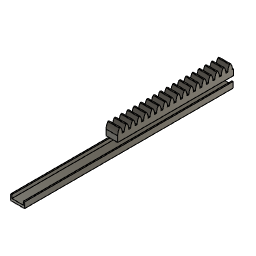
Planar joint (Autodesk Fusion 360 design; units mm, degrees)
Autodesk Fusion 360 part; units mm, degrees
sketch "Sketch1" plane through (0, 0, 0) normal (1, 0, 0) x (0, 1, 0)
  line L0 (0, 0) -> (200, 0)
  line L1 (200, 0) -> (200, 10)
  line L2 (0, 10) -> (0, 0)
  line L3 (0, 15) -> (200, 15.0001) construction
  arc A0 (3.0334, 20) -> (0, 10) centre (18, 10) ccw
  line L4 (3.0334, 20) -> (5.0334, 20)
  line L5 (4.0334, 20) -> (4.0334, 10) construction
  arc A1 (8.0667, 10) -> (5.0334, 20) centre (-9.9333, 10) ccw
  line L6 (14.2098, 20) -> (16.2098, 20)
  line L7 (15.2098, 20) -> (15.2098, 10) construction
  arc A2 (14.2098, 20) -> (11.1765, 10) centre (29.1765, 10) ccw
  arc A3 (19.2432, 10) -> (16.2098, 20) centre (1.2432, 10) ccw
  line L8 (25.3863, 20) -> (27.3863, 20)
  line L9 (26.3863, 20) -> (26.3863, 10) construction
  arc A4 (25.3863, 20) -> (22.3529, 10) centre (40.3529, 10) ccw
  arc A5 (30.4197, 10) -> (27.3863, 20) centre (12.4197, 10) ccw
  line L10 (36.5628, 20) -> (38.5628, 20)
  line L11 (37.5628, 20) -> (37.5628, 10) construction
  arc A6 (36.5628, 20) -> (33.5294, 10) centre (51.5294, 10) ccw
  arc A7 (41.5961, 10) -> (38.5628, 20) centre (23.5961, 10) ccw
  line L12 (47.7392, 20) -> (49.7392, 20)
  line L13 (48.7392, 20) -> (48.7392, 10) construction
  arc A8 (47.7392, 20) -> (44.7059, 10) centre (62.7059, 10) ccw
  arc A9 (52.7726, 10) -> (49.7392, 20) centre (34.7726, 10) ccw
  line L14 (58.9157, 20) -> (60.9157, 20)
  line L15 (59.9157, 20) -> (59.9157, 10) construction
  arc A10 (58.9157, 20) -> (55.8823, 10) centre (73.8823, 10) ccw
  arc A11 (63.9491, 10) -> (60.9157, 20) centre (45.9491, 10) ccw
  line L16 (70.0922, 20) -> (72.0922, 20)
  line L17 (71.0922, 20) -> (71.0922, 10) construction
  arc A12 (70.0922, 20) -> (67.0588, 10) centre (85.0588, 10) ccw
  arc A13 (75.1255, 10) -> (72.0922, 20) centre (57.1255, 10) ccw
  line L18 (81.2687, 20) -> (83.2687, 20)
  line L19 (82.2687, 20) -> (82.2687, 10) construction
  arc A14 (81.2687, 20) -> (78.2353, 10) centre (96.2353, 10) ccw
  arc A15 (86.302, 10) -> (83.2687, 20) centre (68.302, 10) ccw
  line L20 (92.4451, 20) -> (94.4451, 20)
  line L21 (93.4451, 20) -> (93.4451, 10) construction
  arc A16 (92.4451, 20) -> (89.4118, 10) centre (107.4118, 10) ccw
  arc A17 (97.4785, 10) -> (94.4451, 20) centre (79.4785, 10) ccw
  line L22 (103.6216, 20) -> (105.6216, 20)
  line L23 (104.6216, 20) -> (104.6216, 10) construction
  arc A18 (103.6216, 20) -> (100.5882, 10) centre (118.5882, 10) ccw
  arc A19 (108.655, 10) -> (105.6216, 20) centre (90.655, 10) ccw
  line L24 (114.7981, 20) -> (116.7981, 20)
  line L25 (115.7981, 20) -> (115.7981, 10) construction
  arc A20 (114.7981, 20) -> (111.7647, 10) centre (129.7647, 10) ccw
  arc A21 (119.8314, 10) -> (116.7981, 20) centre (101.8314, 10) ccw
  line L26 (125.9745, 20) -> (127.9745, 20)
  line L27 (126.9745, 20) -> (126.9745, 10) construction
  arc A22 (125.9745, 20) -> (122.9412, 10) centre (140.9412, 10) ccw
  arc A23 (131.0079, 10) -> (127.9745, 20) centre (113.0079, 10) ccw
  line L28 (137.151, 20) -> (139.151, 20)
  line L29 (138.151, 20) -> (138.151, 10) construction
  arc A24 (137.151, 20) -> (134.1176, 10) centre (152.1176, 10) ccw
  arc A25 (142.1844, 10) -> (139.151, 20) centre (124.1844, 10) ccw
  line L30 (148.3275, 20) -> (150.3275, 20)
  line L31 (149.3275, 20) -> (149.3275, 10) construction
  arc A26 (148.3275, 20) -> (145.2941, 10) centre (163.2941, 10) ccw
  arc A27 (153.3608, 10) -> (150.3275, 20) centre (135.3608, 10) ccw
  line L32 (159.5039, 20) -> (161.5039, 20)
  line L33 (160.5039, 20) -> (160.5039, 10) construction
  arc A28 (159.5039, 20) -> (156.4706, 10) centre (174.4706, 10) ccw
  arc A29 (164.5373, 10) -> (161.5039, 20) centre (146.5373, 10) ccw
  line L34 (170.6804, 20) -> (172.6804, 20)
  line L35 (171.6804, 20) -> (171.6804, 10) construction
  arc A30 (170.6804, 20) -> (167.6471, 10) centre (185.6471, 10) ccw
  arc A31 (175.7138, 10) -> (172.6804, 20) centre (157.7138, 10) ccw
  line L36 (181.8569, 20) -> (183.8569, 20)
  line L37 (182.8569, 20) -> (182.8569, 10) construction
  arc A32 (181.8569, 20) -> (178.8235, 10) centre (196.8235, 10) ccw
  arc A33 (186.8902, 10) -> (183.8569, 20) centre (168.8902, 10) ccw
  line L38 (193.0334, 20) -> (195.0334, 20)
  line L39 (194.0334, 20) -> (194.0334, 10) construction
  arc A34 (193.0334, 20) -> (190, 10) centre (208, 10) ccw
  arc A35 (198.0667, 10) -> (195.0334, 20) centre (180.0667, 10) ccw
  arc A36 (36.5764, 129.9483) -> (33.491, 119.9458) centre (51.4908, 119.8706) ccw
  arc A37 (41.6234, 119.9458) -> (38.5764, 129.9431) centre (23.4014, 119.855) ccw
  line L40 (37.5764, 129.9457) -> (37.5357, 119.9458) construction
  line L41 (36.5764, 129.9483) -> (38.5764, 129.9431)
  line L42 (182.8569, 170) -> (182.8569, 160) construction
  line L43 (181.8569, 170) -> (183.8569, 170)
  arc A38 (186.8902, 160) -> (183.8569, 170) centre (168.8902, 160) ccw
  arc A39 (181.8569, 170) -> (178.8235, 160) centre (196.8235, 160) ccw
  arc A40 (169.119, 168.7106) -> (167.8682, 158.3358) centre (185.5948, 161.4615) ccw
  line L44 (169.119, 168.7106) -> (171.0886, 169.0579)
  arc A41 (175.8124, 159.7366) -> (171.0886, 169.0579) centre (158.0859, 156.6109) ccw
  line L45 (170.1038, 168.8843) -> (171.8403, 159.0362) construction
  arc A42 (156.7986, 165.2289) -> (157.3684, 154.7945) centre (174.2828, 160.9509) ccw
  line L46 (156.7986, 165.2289) -> (158.678, 165.9129)
  arc A43 (164.9486, 157.5535) -> (158.678, 165.9129) centre (148.0341, 151.3971) ccw
  line L47 (157.7383, 165.5709) -> (161.1585, 156.174) construction
  arc A44 (145.2699, 159.6606) -> (147.6429, 149.4837) centre (163.2314, 158.4837) ccw
  line L48 (145.2699, 159.6606) -> (147.002, 160.6606)
  arc A45 (154.6289, 153.5171) -> (147.002, 160.6606) centre (139.0405, 144.5171) ccw
  line L49 (146.1359, 160.1606) -> (151.1359, 151.5004) construction
  arc A46 (134.8833, 152.1751) -> (138.9875, 142.5648) centre (152.7763, 154.135) ccw
  line L50 (134.8833, 152.1751) -> (136.4154, 153.4606)
  arc A47 (145.1669, 147.75) -> (136.4154, 153.4606) centre (131.3781, 136.1798) ccw
  line L51 (135.6493, 152.8179) -> (142.0772, 145.1574) construction
  arc A48 (125.9543, 142.9996) -> (131.665, 134.248) centre (143.2351, 148.0368) ccw
  line L52 (125.9543, 142.9996) -> (127.2399, 144.5317)
  arc A49 (136.8502, 140.4275) -> (127.2399, 144.5317) centre (125.28, 126.6387) ccw
  line L53 (126.5971, 143.7656) -> (134.2576, 137.3378) construction
  arc A50 (118.7543, 132.413) -> (125.8979, 124.786) centre (134.8979, 140.3745) ccw
  line L54 (118.7543, 132.413) -> (119.7543, 134.1451)
  arc A51 (129.9313, 131.772) -> (119.7543, 134.1451) centre (120.9312, 116.1836) ccw
  line L55 (119.2543, 133.279) -> (127.9146, 128.279) construction
  arc A52 (113.502, 120.737) -> (121.8615, 114.4664) centre (128.0178, 131.3808) ccw
  line L56 (113.502, 120.737) -> (114.1861, 122.6164)
  arc A53 (124.6205, 122.0466) -> (114.1861, 122.6164) centre (118.4641, 105.1322) ccw
  line L57 (113.8441, 121.6767) -> (123.241, 118.2565) construction
  arc A54 (110.3571, 108.3263) -> (119.6784, 103.6026) centre (122.8041, 121.3291) ccw
  line L58 (110.3571, 108.3263) -> (110.7044, 110.2959)
  arc A55 (121.0792, 111.5467) -> (110.7044, 110.2959) centre (117.9535, 93.8202) ccw
  line L59 (110.5307, 109.3111) -> (120.3788, 107.5747) construction
  arc A56 (109.415, 95.5581) -> (119.415, 92.5247) centre (119.415, 110.5247) ccw
  line L60 (109.415, 95.5581) -> (109.415, 97.5581)
  arc A57 (119.415, 100.5914) -> (109.415, 97.5581) centre (119.415, 82.5914) ccw
  line L61 (109.415, 96.5581) -> (119.415, 96.5581) construction
  arc A58 (110.7044, 82.8202) -> (121.0792, 81.5694) centre (117.9535, 99.296) ccw
  line L62 (110.7044, 82.8202) -> (110.3571, 84.7898)
  arc A59 (119.6784, 89.5136) -> (110.3571, 84.7898) centre (122.8041, 71.7871) ccw
  line L63 (110.5307, 83.805) -> (120.3788, 85.5415) construction
  arc A60 (114.1861, 70.4998) -> (124.6205, 71.0695) centre (118.4641, 87.984) ccw
  line L64 (114.1861, 70.4998) -> (113.502, 72.3792)
  arc A61 (121.8615, 78.6498) -> (113.502, 72.3792) centre (128.0178, 61.7353) ccw
  line L65 (113.8441, 71.4395) -> (123.241, 74.8597) construction
  arc A62 (119.7543, 58.9711) -> (129.9313, 61.3441) centre (120.9312, 76.9326) ccw
  line L66 (119.7543, 58.9711) -> (118.7543, 60.7031)
  arc A63 (125.8979, 68.3301) -> (118.7543, 60.7031) centre (134.8979, 52.7417) ccw
  line L67 (119.2543, 59.8371) -> (127.9146, 64.8371) construction
  arc A64 (127.2399, 48.5845) -> (136.8502, 52.6887) centre (125.28, 66.4775) ccw
  line L68 (127.2399, 48.5845) -> (125.9543, 50.1166)
  arc A65 (131.665, 58.8681) -> (125.9543, 50.1166) centre (143.2351, 45.0793) ccw
  line L69 (126.5971, 49.3505) -> (134.2576, 55.7784) construction
  arc A66 (136.4154, 39.6555) -> (145.1669, 45.3662) centre (131.3781, 56.9363) ccw
  line L70 (136.4154, 39.6555) -> (134.8833, 40.9411)
  arc A67 (138.9875, 50.5513) -> (134.8833, 40.9411) centre (152.7763, 38.9812) ccw
  line L71 (135.6493, 40.2983) -> (142.0772, 47.9588) construction
  arc A68 (147.002, 32.4555) -> (154.6289, 39.5991) centre (139.0405, 48.5991) ccw
  line L72 (147.002, 32.4555) -> (145.2699, 33.4555)
  arc A69 (147.6429, 43.6325) -> (145.2699, 33.4555) centre (163.2314, 34.6324) ccw
  line L73 (146.1359, 32.9555) -> (151.1359, 41.6158) construction
  arc A70 (158.678, 27.2032) -> (164.9486, 35.5627) centre (148.0341, 41.719) ccw
  line L74 (158.678, 27.2032) -> (156.7986, 27.8873)
  arc A71 (157.3684, 38.3217) -> (156.7986, 27.8873) centre (174.2828, 32.1653) ccw
  line L75 (157.7383, 27.5453) -> (161.1585, 36.9422) construction
  arc A72 (171.0886, 24.0583) -> (175.8124, 33.3796) centre (158.0859, 36.5053) ccw
  line L76 (171.0886, 24.0583) -> (169.119, 24.4056)
  arc A73 (167.8682, 34.7804) -> (169.119, 24.4056) centre (185.5948, 31.6547) ccw
  line L77 (170.1038, 24.2319) -> (171.8403, 34.08) construction
  arc A74 (183.8569, 23.1162) -> (186.8902, 33.1162) centre (168.8902, 33.1162) ccw
  line L78 (183.8569, 23.1162) -> (181.8569, 23.1162)
  arc A75 (178.8235, 33.1162) -> (181.8569, 23.1162) centre (196.8235, 33.1162) ccw
  line L79 (182.8569, 23.1162) -> (182.8569, 33.1162) construction
  arc A76 (196.5947, 24.4056) -> (197.8455, 34.7804) centre (180.119, 31.6547) ccw
  line L80 (196.5947, 24.4056) -> (194.6251, 24.0583)
  arc A77 (189.9014, 33.3796) -> (194.6251, 24.0583) centre (207.6279, 36.5053) ccw
  line L81 (195.6099, 24.2319) -> (193.8735, 34.08) construction
  arc A78 (208.9152, 27.8873) -> (208.3454, 38.3217) centre (191.431, 32.1653) ccw
  line L82 (208.9152, 27.8873) -> (207.0358, 27.2032)
  arc A79 (200.7652, 35.5627) -> (207.0358, 27.2032) centre (217.6796, 41.719) ccw
  line L83 (207.9755, 27.5453) -> (204.5553, 36.9422) construction
  arc A80 (220.4439, 33.4555) -> (218.0708, 43.6325) centre (202.4824, 34.6324) ccw
  line L84 (220.4439, 33.4555) -> (218.7118, 32.4555)
  arc A81 (211.0848, 39.5991) -> (218.7118, 32.4555) centre (226.6733, 48.5991) ccw
  line L85 (219.5778, 32.9555) -> (214.5778, 41.6158) construction
  arc A82 (230.8305, 40.9411) -> (226.7263, 50.5513) centre (212.9375, 38.9812) ccw
  line L86 (230.8305, 40.9411) -> (229.2984, 39.6555)
  arc A83 (220.5468, 45.3662) -> (229.2984, 39.6555) centre (234.3356, 56.9363) ccw
  line L87 (230.0644, 40.2983) -> (223.6366, 47.9588) construction
  arc A84 (239.7594, 50.1166) -> (234.0488, 58.8681) centre (222.4786, 45.0793) ccw
  line L88 (239.7594, 50.1166) -> (238.4739, 48.5845)
  arc A85 (228.8636, 52.6887) -> (238.4739, 48.5845) centre (240.4338, 66.4775) ccw
  line L89 (239.1167, 49.3505) -> (231.4562, 55.7784) construction
  arc A86 (246.9595, 60.7031) -> (239.8159, 68.3301) centre (230.8159, 52.7417) ccw
  line L90 (246.9595, 60.7031) -> (245.9595, 58.9711)
  arc A87 (235.7825, 61.3441) -> (245.9595, 58.9711) centre (244.7825, 76.9326) ccw
  line L91 (246.4595, 59.8371) -> (237.7992, 64.8371) construction
  arc A88 (252.2117, 72.3792) -> (243.8523, 78.6498) centre (237.6959, 61.7353) ccw
  line L92 (252.2117, 72.3792) -> (251.5277, 70.4998)
  arc A89 (241.0933, 71.0695) -> (251.5277, 70.4998) centre (247.2497, 87.984) ccw
  line L93 (251.8697, 71.4395) -> (242.4728, 74.8597) construction
  arc A90 (255.3567, 84.7898) -> (246.0354, 89.5136) centre (242.9097, 71.7871) ccw
  line L94 (255.3567, 84.7898) -> (255.0094, 82.8202)
  arc A91 (244.6346, 81.5694) -> (255.0094, 82.8202) centre (247.7603, 99.296) ccw
  line L95 (255.1831, 83.805) -> (245.335, 85.5415) construction
  arc A92 (256.2988, 97.5581) -> (246.2988, 100.5914) centre (246.2988, 82.5914) ccw
  line L96 (256.2988, 97.5581) -> (256.2988, 95.5581)
  arc A93 (246.2988, 92.5247) -> (256.2988, 95.5581) centre (246.2988, 110.5247) ccw
  line L97 (256.2988, 96.5581) -> (246.2988, 96.5581) construction
  arc A94 (255.0094, 110.2959) -> (244.6346, 111.5467) centre (247.7603, 93.8202) ccw
  line L98 (255.0094, 110.2959) -> (255.3567, 108.3263)
  arc A95 (246.0354, 103.6026) -> (255.3567, 108.3263) centre (242.9097, 121.3291) ccw
  line L99 (255.1831, 109.3111) -> (245.335, 107.5747) construction
  arc A96 (251.5277, 122.6164) -> (241.0933, 122.0466) centre (247.2497, 105.1322) ccw
  line L100 (251.5277, 122.6164) -> (252.2117, 120.737)
  arc A97 (243.8523, 114.4664) -> (252.2117, 120.737) centre (237.6959, 131.3808) ccw
  line L101 (251.8697, 121.6767) -> (242.4728, 118.2565) construction
  arc A98 (245.9595, 134.1451) -> (235.7825, 131.772) centre (244.7825, 116.1836) ccw
  line L102 (245.9595, 134.1451) -> (246.9595, 132.413)
  arc A99 (239.8159, 124.786) -> (246.9595, 132.413) centre (230.8159, 140.3745) ccw
  line L103 (246.4595, 133.279) -> (237.7992, 128.279) construction
  arc A100 (238.4739, 144.5317) -> (228.8636, 140.4275) centre (240.4338, 126.6387) ccw
  line L104 (238.4739, 144.5317) -> (239.7594, 142.9996)
  arc A101 (234.0488, 134.248) -> (239.7594, 142.9996) centre (222.4786, 148.0368) ccw
  line L105 (239.1167, 143.7656) -> (231.4562, 137.3378) construction
  arc A102 (229.2984, 153.4606) -> (220.5468, 147.75) centre (234.3356, 136.1798) ccw
  line L106 (229.2984, 153.4606) -> (230.8305, 152.1751)
  arc A103 (226.7263, 142.5648) -> (230.8305, 152.1751) centre (212.9375, 154.135) ccw
  line L107 (230.0644, 152.8179) -> (223.6366, 145.1574) construction
  arc A104 (218.7118, 160.6606) -> (211.0848, 153.5171) centre (226.6733, 144.5171) ccw
  line L108 (218.7118, 160.6606) -> (220.4439, 159.6606)
  arc A105 (218.0708, 149.4837) -> (220.4439, 159.6606) centre (202.4824, 158.4837) ccw
  line L109 (219.5778, 160.1606) -> (214.5778, 151.5004) construction
  arc A106 (207.0358, 165.9129) -> (200.7652, 157.5535) centre (217.6796, 151.3971) ccw
  line L110 (207.0358, 165.9129) -> (208.9152, 165.2289)
  arc A107 (208.3454, 154.7945) -> (208.9152, 165.2289) centre (191.431, 160.9509) ccw
  line L111 (207.9755, 165.5709) -> (204.5553, 156.174) construction
  arc A108 (194.6251, 169.0579) -> (189.9014, 159.7366) centre (207.6279, 156.6109) ccw
  line L112 (194.6251, 169.0579) -> (196.5947, 168.7106)
  arc A109 (197.8455, 158.3358) -> (196.5947, 168.7106) centre (180.119, 161.4615) ccw
  line L113 (195.6099, 168.8843) -> (193.8735, 159.0362) construction
  arc A110 (167.8682, 158.3358) -> (164.9486, 157.5535) centre (182.8569, 96.5581) ccw
  arc A111 (157.3684, 154.7945) -> (154.6289, 153.5171) centre (182.8569, 96.5581) ccw
  arc A112 (147.6429, 149.4837) -> (145.1669, 147.75) centre (182.8569, 96.5581) ccw
  arc A113 (138.9875, 142.5648) -> (136.8502, 140.4275) centre (182.8569, 96.5581) ccw
  arc A114 (131.665, 134.248) -> (129.9313, 131.772) centre (182.8569, 96.5581) ccw
  arc A115 (125.8979, 124.786) -> (124.6205, 122.0466) centre (182.8569, 96.5581) ccw
  arc A116 (121.8615, 114.4664) -> (121.0792, 111.5467) centre (182.8569, 96.5581) ccw
  arc A117 (119.6784, 103.6026) -> (119.415, 100.5914) centre (182.8569, 96.5581) ccw
  arc A118 (119.415, 92.5247) -> (119.6784, 89.5136) centre (182.8569, 96.5581) ccw
  arc A119 (121.0792, 81.5694) -> (121.8615, 78.6498) centre (182.8569, 96.5581) ccw
  arc A120 (124.6205, 71.0695) -> (125.8979, 68.3301) centre (182.8569, 96.5581) ccw
  arc A121 (129.9313, 61.3441) -> (131.665, 58.8681) centre (182.8569, 96.5581) ccw
  arc A122 (136.8502, 52.6887) -> (138.9875, 50.5513) centre (182.8569, 96.5581) ccw
  arc A123 (145.1669, 45.3662) -> (147.6429, 43.6325) centre (182.8569, 96.5581) ccw
  arc A124 (154.6289, 39.5991) -> (157.3684, 38.3217) centre (182.8569, 96.5581) ccw
  arc A125 (164.9486, 35.5627) -> (167.8682, 34.7804) centre (182.8569, 96.5581) ccw
  arc A126 (175.8124, 33.3796) -> (178.8235, 33.1162) centre (182.8569, 96.5581) ccw
  arc A127 (186.8902, 33.1162) -> (189.9014, 33.3796) centre (182.8569, 96.5581) ccw
  arc A128 (197.8455, 34.7804) -> (200.7652, 35.5627) centre (182.8569, 96.5581) ccw
  arc A129 (208.3454, 38.3217) -> (211.0848, 39.5991) centre (182.8569, 96.5581) ccw
  arc A130 (218.0708, 43.6325) -> (220.5468, 45.3662) centre (182.8569, 96.5581) ccw
  arc A131 (226.7263, 50.5513) -> (228.8636, 52.6887) centre (182.8569, 96.5581) ccw
  arc A132 (234.0488, 58.8681) -> (235.7825, 61.3441) centre (182.8569, 96.5581) ccw
  arc A133 (239.8159, 68.3301) -> (241.0933, 71.0695) centre (182.8569, 96.5581) ccw
  arc A134 (243.8523, 78.6498) -> (244.6346, 81.5694) centre (182.8569, 96.5581) ccw
  arc A135 (246.0354, 89.5136) -> (246.2988, 92.5247) centre (182.8569, 96.5581) ccw
  arc A136 (246.2988, 100.5914) -> (246.0354, 103.6026) centre (182.8569, 96.5581) ccw
  arc A137 (244.6346, 111.5467) -> (243.8523, 114.4664) centre (182.8569, 96.5581) ccw
  arc A138 (241.0933, 122.0466) -> (239.8159, 124.786) centre (182.8569, 96.5581) ccw
  arc A139 (235.7825, 131.772) -> (234.0488, 134.248) centre (182.8569, 96.5581) ccw
  arc A140 (228.8636, 140.4275) -> (226.7263, 142.5648) centre (182.8569, 96.5581) ccw
  arc A141 (220.5468, 147.75) -> (218.0708, 149.4837) centre (182.8569, 96.5581) ccw
  arc A142 (211.0848, 153.5171) -> (208.3454, 154.7945) centre (182.8569, 96.5581) ccw
  arc A143 (200.7652, 157.5535) -> (197.8455, 158.3358) centre (182.8569, 96.5581) ccw
  arc A144 (189.9014, 159.7366) -> (186.8902, 160) centre (182.8569, 96.5581) ccw
  arc A145 (178.8235, 160) -> (175.8124, 159.7366) centre (182.8569, 96.5581) ccw
  line L114 (11.1765, 10) -> (8.0667, 10)
  line L115 (22.3529, 10) -> (19.2432, 10)
  line L116 (33.5294, 10) -> (30.4197, 10)
  line L117 (44.7059, 10) -> (41.5961, 10)
  line L118 (55.8823, 10) -> (52.7726, 10)
  line L119 (67.0588, 10) -> (63.9491, 10)
  line L120 (78.2353, 10) -> (75.1255, 10)
  line L121 (89.4118, 10) -> (86.302, 10)
  line L122 (100.5882, 10) -> (97.4785, 10)
  line L123 (111.7647, 10) -> (108.655, 10)
  line L124 (122.9412, 10) -> (119.8314, 10)
  line L125 (134.1176, 10) -> (131.0079, 10)
  line L126 (145.2941, 10) -> (142.1844, 10)
  line L127 (156.4706, 10) -> (153.3608, 10)
  line L128 (167.6471, 10) -> (164.5373, 10)
  line L129 (178.8235, 10) -> (175.7138, 10)
  line L130 (200, 10) -> (198.0667, 10)
  line L131 (190, 10) -> (186.8902, 10)
  circle A146 centre (182.8569, 96.5581) radius 10
  arc A147 (212.3042, 133.5512) -> (182.8569, 143.8405) centre (182.8569, 96.5581) ccw
  arc A148 (206.153, 125.8239) -> (212.3042, 133.5512) centre (209.2286, 129.6875) ccw
  arc A149 (206.153, 125.8239) -> (182.8569, 133.9639) centre (182.8569, 96.5581) ccw
  arc A150 (182.8569, 143.8405) -> (182.8569, 133.9639) centre (182.8569, 138.9022) ccw
  arc A151 (209.2286, 129.6875) -> (182.8569, 138.9022) centre (182.8569, 96.5581) ccw construction
  arc A152 (145.8639, 102.1003) -> (136.0963, 103.5636) centre (140.9801, 102.8319) ccw
  arc A153 (145.8639, 102.1003) -> (150.4625, 77.8552) centre (182.8569, 96.5581) ccw
  arc A154 (141.9091, 72.9169) -> (150.4625, 77.8552) centre (146.1858, 75.386) ccw
  arc A155 (140.9801, 102.8319) -> (146.1858, 75.386) centre (182.8569, 96.5581) ccw construction
  arc A156 (136.0963, 103.5636) -> (141.9091, 72.9169) centre (182.8569, 96.5581) ccw
  arc A157 (196.5537, 61.7501) -> (200.1702, 52.5595) centre (198.362, 57.1548) ccw
  arc A158 (196.5537, 61.7501) -> (215.2513, 77.8552) centre (182.8569, 96.5581) ccw
  arc A159 (223.8047, 72.9169) -> (215.2513, 77.8552) centre (219.528, 75.386) ccw
  arc A160 (198.362, 57.1548) -> (219.528, 75.386) centre (182.8569, 96.5581) ccw construction
  arc A161 (200.1702, 52.5595) -> (223.8047, 72.9169) centre (182.8569, 96.5581) ccw
  arc A162 (128.1606, 138.2003) -> (125.0188, 133.7133) centre (182.8569, 96.5581) ccw construction
  arc A163 (31.6681, 119.5948) -> (25.0272, 127.6651) centre (14.8679, 112.5377) ccw
  line L132 (24.1023, 127.2848) -> (27.8915, 118.0306) construction
  arc A164 (23.1774, 126.9046) -> (24.1546, 116.4827) centre (40.8131, 123.3014) ccw
  line L133 (23.1774, 126.9046) -> (25.0272, 127.6651)
  arc A165 (22.6048, 115.4609) -> (13.3811, 120.3754) centre (9.7841, 102.5117) ccw
  line L134 (12.6721, 119.6702) -> (19.7143, 112.5704) construction
  arc A166 (11.9631, 118.965) -> (16.8543, 109.7103) centre (29.6353, 122.385) ccw
  line L135 (11.9631, 118.965) -> (13.3811, 120.3754)
  arc A167 (15.8134, 108.1732) -> (5.4111, 109.1839) centre (8.9241, 91.3035) ccw
  line L136 (5.026, 108.2611) -> (14.2491, 104.3967) construction
  arc A168 (4.6409, 107.3382) -> (12.7013, 100.6598) centre (19.659, 117.2607) ccw
  line L137 (4.6409, 107.3382) -> (5.4111, 109.1839)
  arc A169 (12.3279, 98.8413) -> (2.3306, 95.7943) centre (12.4187, 80.6193) ccw
  line L138 (2.328, 94.7943) -> (12.3279, 94.7536) construction
  arc A170 (2.3253, 93.7943) -> (12.3279, 90.7089) centre (12.4031, 108.7087) ccw
  line L139 (2.3253, 93.7943) -> (2.3306, 95.7943)
  arc A171 (12.6788, 88.886) -> (4.6086, 82.2451) centre (19.736, 72.0858) ccw
  line L140 (4.9888, 81.3202) -> (14.2431, 85.1094) construction
  arc A172 (5.3691, 80.3953) -> (15.791, 81.3725) centre (8.9722, 98.031) ccw
  line L141 (5.3691, 80.3953) -> (4.6086, 82.2451)
  arc A173 (16.8128, 79.8227) -> (11.8982, 70.599) centre (29.7619, 67.002) ccw
  line L142 (12.6035, 69.89) -> (19.7032, 76.9322) construction
  arc A174 (13.3087, 69.181) -> (22.5633, 74.0722) centre (9.8887, 86.8532) ccw
  line L143 (13.3087, 69.181) -> (11.8982, 70.599)
  arc A175 (24.1005, 73.0313) -> (23.0897, 62.629) centre (40.9702, 66.142) ccw
  line L144 (24.0126, 62.2439) -> (27.877, 71.467) construction
  arc A176 (24.9355, 61.8588) -> (31.6139, 69.9192) centre (15.013, 76.8769) ccw
  line L145 (24.9355, 61.8588) -> (23.0897, 62.629)
  arc A177 (33.4323, 69.5458) -> (36.4793, 59.5485) centre (51.6544, 69.6366) ccw
  line L146 (37.4793, 59.5459) -> (37.52, 69.5458) construction
  arc A178 (38.4793, 59.5432) -> (41.5648, 69.5458) centre (23.565, 69.621) ccw
  line L147 (38.4793, 59.5432) -> (36.4793, 59.5485)
  arc A179 (43.3877, 69.8967) -> (50.0286, 61.8265) centre (60.1879, 76.9539) ccw
  line L148 (50.9535, 62.2067) -> (47.1642, 71.461) construction
  arc A180 (51.8783, 62.587) -> (50.9011, 73.0089) centre (34.2427, 66.1901) ccw
  line L149 (51.8783, 62.587) -> (50.0286, 61.8265)
  arc A181 (52.451, 74.0307) -> (61.6747, 69.1161) centre (65.2717, 86.9798) ccw
  line L150 (62.3837, 69.8214) -> (55.3414, 76.9211) construction
  arc A182 (63.0926, 70.5266) -> (58.2015, 79.7812) centre (45.4205, 67.1066) ccw
  line L151 (63.0926, 70.5266) -> (61.6747, 69.1161)
  arc A183 (59.2423, 81.3184) -> (69.6447, 80.3076) centre (66.1317, 98.1881) ccw
  line L152 (70.0298, 81.2305) -> (60.8066, 85.0949) construction
  arc A184 (70.4149, 82.1534) -> (62.3545, 88.8318) centre (55.3968, 72.2309) ccw
  line L153 (70.4149, 82.1534) -> (69.6447, 80.3076)
  arc A185 (62.7279, 90.6502) -> (72.7252, 93.6972) centre (62.6371, 108.8723) ccw
  line L154 (72.7278, 94.6972) -> (62.7279, 94.7379) construction
  arc A186 (72.7304, 95.6972) -> (62.7279, 98.7827) centre (62.6527, 80.7829) ccw
  line L155 (72.7304, 95.6972) -> (72.7252, 93.6972)
  arc A187 (62.3769, 100.6056) -> (70.4472, 107.2465) centre (55.3198, 117.4058) ccw
  line L156 (70.0669, 108.1714) -> (60.8127, 104.3821) construction
  arc A188 (69.6867, 109.0962) -> (59.2648, 108.119) centre (66.0835, 91.4606) ccw
  line L157 (69.6867, 109.0962) -> (70.4472, 107.2465)
  arc A189 (58.243, 109.6689) -> (63.1575, 118.8926) centre (45.2938, 122.4896) ccw
  line L158 (62.4523, 119.6016) -> (55.3525, 112.5593) construction
  arc A190 (61.7471, 120.3105) -> (52.4924, 115.4194) centre (65.1671, 102.6384) ccw
  line L159 (61.7471, 120.3105) -> (63.1575, 118.8926)
  arc A191 (50.9553, 116.4602) -> (51.966, 126.8626) centre (34.0856, 123.3496) ccw
  line L160 (51.0432, 127.2477) -> (47.1788, 118.0245) construction
  arc A192 (50.1203, 127.6328) -> (43.4419, 119.5724) centre (60.0428, 112.6147) ccw
  line L161 (50.1203, 127.6328) -> (51.966, 126.8626)
  arc A193 (16.8476, 109.7171) -> (15.8134, 108.1732) centre (37.5279, 94.7458) ccw
  arc A194 (12.6925, 100.6634) -> (12.3279, 98.8413) centre (37.5279, 94.7458) ccw
  arc A195 (12.3184, 90.7089) -> (12.6788, 88.886) centre (37.5279, 94.7458) ccw
  arc A196 (15.7822, 81.369) -> (16.8128, 79.8227) centre (37.5279, 94.7458) ccw
  arc A197 (22.5566, 74.0655) -> (24.1005, 73.0313) centre (37.5279, 94.7458) ccw
  arc A198 (31.6102, 69.9104) -> (33.4323, 69.5458) centre (37.5279, 94.7458) ccw
  arc A199 (41.5648, 69.5363) -> (43.3877, 69.8967) centre (37.5279, 94.7458) ccw
  arc A200 (50.9047, 73.0001) -> (52.451, 74.0307) centre (37.5279, 94.7458) ccw
  arc A201 (58.2082, 79.7745) -> (59.2423, 81.3184) centre (37.5279, 94.7458) ccw
  arc A202 (62.3632, 88.8281) -> (62.7279, 90.6502) centre (37.5279, 94.7458) ccw
  arc A203 (62.7374, 98.7827) -> (62.3769, 100.6056) centre (37.5279, 94.7458) ccw
  arc A204 (59.2735, 108.1226) -> (58.243, 109.6689) centre (37.5279, 94.7458) ccw
  arc A205 (52.4992, 115.4261) -> (50.9553, 116.4602) centre (37.5279, 94.7458) ccw
  arc A206 (43.4455, 119.5811) -> (41.6234, 119.9458) centre (37.5279, 94.7458) ccw
  arc A207 (33.491, 119.9552) -> (31.6681, 119.5948) centre (37.5279, 94.7458) ccw
  arc A208 (24.1511, 116.4914) -> (22.6048, 115.4609) centre (37.5279, 94.7458) ccw
  arc A209 (54.1562, 96.2405) -> (37.5279, 111.4411) centre (37.5279, 94.7458) ccw
  arc A210 (49.1534, 95.7908) -> (54.1562, 96.2405) centre (51.6548, 96.0157) ccw
  arc A211 (49.1534, 95.7908) -> (37.5279, 106.4182) centre (37.5279, 94.7458) ccw
  arc A212 (37.5279, 111.4411) -> (37.5279, 106.4182) centre (37.5279, 108.9297) ccw
  arc A213 (51.6548, 96.0157) -> (37.5279, 108.9297) centre (37.5279, 94.7458) ccw construction
  arc A214 (30.8101, 104.2913) -> (27.4193, 88.9096) centre (37.5279, 94.7458) ccw
  arc A215 (23.0693, 86.3981) -> (27.4193, 88.9096) centre (25.2443, 87.6538) ccw
  arc A216 (27.9193, 108.399) -> (23.0693, 86.3981) centre (37.5279, 94.7458) ccw
  arc A217 (29.3647, 106.3451) -> (25.2443, 87.6538) centre (37.5279, 94.7458) ccw construction
  arc A218 (30.8101, 104.2913) -> (27.9193, 108.399) centre (29.3647, 106.3451) ccw
  arc A219 (32.6201, 84.1553) -> (47.6365, 88.9096) centre (37.5279, 94.7458) ccw
  arc A220 (51.9865, 86.3981) -> (47.6365, 88.9096) centre (49.8115, 87.6538) ccw
  arc A221 (30.5082, 79.5979) -> (51.9865, 86.3981) centre (37.5279, 94.7458) ccw
  arc A222 (31.5642, 81.8766) -> (49.8115, 87.6538) centre (37.5279, 94.7458) ccw construction
  arc A223 (32.6201, 84.1553) -> (30.5082, 79.5979) centre (31.5642, 81.8766) ccw
  circle A224 centre (37.5279, 94.7458) radius 5
  point P0 (11.1765, 15)
  point P1 (22.3529, 15)
  point P2 (33.5294, 15)
  point P3 (44.7059, 15)
  point P4 (55.8823, 15)
  point P5 (67.0588, 15)
  point P6 (78.2353, 15)
  point P7 (89.4118, 15)
  point P8 (100.5882, 15)
  point P9 (111.7647, 15)
  point P10 (122.9412, 15)
  point P11 (134.1176, 15)
  point P12 (145.2941, 15)
  point P13 (156.4706, 15)
  point P14 (167.6471, 15)
  point P15 (178.8235, 15)
  point P16 (190, 15)
  point P17 (185.6471, 160)
  point P18 (180.0667, 160)
  point P19 (174.5881, 159.5207)
  point P20 (169.0925, 158.5517)
  point P21 (163.7804, 157.1283)
  point P22 (158.5366, 155.2197)
  point P23 (153.5523, 152.8955)
  point P24 (148.7196, 150.1053)
  point P25 (144.2146, 146.9509)
  point P26 (139.9398, 143.3639)
  point P27 (136.051, 139.4752)
  point P28 (132.4641, 135.2004)
  point P29 (129.3096, 130.6954)
  point P30 (126.5195, 125.8627)
  point P31 (124.1953, 120.8784)
  point P32 (122.2867, 115.6346)
  point P33 (120.8633, 110.3224)
  point P34 (119.8943, 104.8269)
  point P35 (119.415, 99.3482)
  point P36 (119.415, 93.7679)
  point P37 (119.8943, 88.2893)
  point P38 (120.8633, 82.7937)
  point P39 (122.2867, 77.4816)
  point P40 (124.1953, 72.2378)
  point P41 (126.5195, 67.2535)
  point P42 (129.3096, 62.4208)
  point P43 (132.4641, 57.9158)
  point P44 (136.051, 53.641)
  point P45 (139.9398, 49.7522)
  point P46 (144.2146, 46.1653)
  point P47 (148.7196, 43.0108)
  point P48 (153.5523, 40.2207)
  point P49 (158.5366, 37.8965)
  point P50 (163.7804, 35.9879)
  point P51 (169.0925, 34.5645)
  point P52 (174.5881, 33.5955)
  point P53 (180.0667, 33.1162)
  point P54 (185.6471, 33.1162)
  point P55 (191.1257, 33.5955)
  point P56 (196.6212, 34.5645)
  point P57 (201.9334, 35.9879)
  point P58 (207.1772, 37.8965)
  point P59 (212.1615, 40.2207)
  point P60 (216.9942, 43.0108)
  point P61 (221.4992, 46.1653)
  point P62 (225.774, 49.7522)
  point P63 (229.6627, 53.641)
  point P64 (233.2497, 57.9158)
  point P65 (236.4041, 62.4208)
  point P66 (239.1943, 67.2535)
  point P67 (241.5185, 72.2378)
  point P68 (243.4271, 77.4816)
  point P69 (244.8505, 82.7937)
  point P70 (245.8195, 88.2893)
  point P71 (246.2988, 93.7679)
  point P72 (246.2988, 99.3482)
  point P73 (245.8195, 104.8269)
  point P74 (244.8505, 110.3224)
  point P75 (243.4271, 115.6346)
  point P76 (241.5185, 120.8784)
  point P77 (239.1943, 125.8627)
  point P78 (236.4041, 130.6954)
  point P79 (233.2497, 135.2004)
  point P80 (229.6627, 139.4752)
  point P81 (225.774, 143.3639)
  point P82 (221.4992, 146.9509)
  point P83 (216.9942, 150.1053)
  point P84 (212.1615, 152.8955)
  point P85 (207.1772, 155.2197)
  point P86 (201.9334, 157.1283)
  point P87 (196.6212, 158.5517)
  point P88 (191.1257, 159.5207)
  point P89 (37.5279, 94.7458)
  point P90 (37.5279, 94.7458)
  point P91 (37.5279, 94.7458)
  point P92 (37.5279, 94.7458)
  point P93 (37.5279, 94.7458)
  point P94 (37.5279, 94.7458)
  point P95 (37.5279, 94.7458)
  point P96 (37.5279, 94.7458)
  point P97 (37.5279, 94.7458)
  point P98 (37.5279, 94.7458)
  point P99 (37.5279, 94.7458)
  point P100 (37.5279, 94.7458)
  point P101 (37.5279, 94.7458)
  point P102 (37.5279, 94.7458)
  point P103 (37.5279, 94.7458)
  point P104 (37.5279, 94.7458)
  point P105 (37.5279, 94.7458)
  point P106 (37.5279, 94.7458)
  point P107 (37.5279, 94.7458)
  point P108 (37.5279, 94.7458)
  point P109 (37.5279, 94.7458)
  point P110 (37.5279, 94.7458)
  point P111 (37.5279, 94.7458)
  point P112 (37.5279, 94.7458)
  point P113 (37.5279, 94.7458)
  point P114 (37.5279, 94.7458)
  point P115 (37.5279, 94.7458)
  point P116 (37.5279, 94.7458)
  point P117 (37.5279, 94.7458)
  point P118 (37.5279, 94.7458)
  point P119 (37.5279, 94.7458)
  point P120 (37.5279, 94.7458)
  point P121 (37.5279, 94.7458)
  dimension "d1" = 5
  dimension "d2" = 10
  dimension "d3" = 10
  dimension "d4" = 200
  dimension "d5" = 18
  dimension "d6" = 2
  dimension "d9" = -190
  dimension "d10" = 0
  dimension "d12" = 2
  dimension "d14" = 18
  dimension "d16" = 10
  dimension "d19" = 127.14
  dimension "d20" = 18
  dimension "d21" = 18
  dimension "d22" = 2
  dimension "d23" = 10
  dimension "d25" = 360
  dimension "d38" = 20
  dimension "d40" = 360
  dimension "d92" = 25.2
  dimension "d94" = 360
  dimension "d96" = 360
  dimension "d97" = 10
  constraint horizontal L0
  constraint vertical L1
  constraint horizontal L130
  constraint vertical L2
  constraint coincident L0.start L2.end
  constraint perpendicular L2 L3
  constraint vertical L1.end L3.end
  constraint vertical L2.start L3.start
  constraint tangent L2 A0
  constraint horizontal L4
  constraint midpoint L4 L5.start
  constraint perpendicular L5 L130
  constraint symmetric L2.start L5 A1.start
  constraint symmetric A0.start L4.end L5
  constraint symmetric A0 L5 A1
  constraint vertical A110.centre L42.end
  constraint horizontal L42.end A39.end
  constraint horizontal A38.start L42.end
  constraint horizontal L43
  constraint coincident A38.start A111
  constraint concentric A110 A111
  constraint concentric A111 A112
  constraint concentric A112 A113
  constraint concentric A113 A114
  constraint concentric A114 A115
  constraint concentric A115 A116
  constraint concentric A116 A117
  constraint concentric A117 A118
  constraint concentric A118 A119
  constraint concentric A119 A120
  constraint concentric A120 A121
  constraint concentric A121 A122
  constraint concentric A122 A123
  constraint concentric A123 A124
  constraint concentric A124 A125
  constraint concentric A125 A126
  constraint concentric A126 A127
  constraint concentric A127 A128
  constraint concentric A128 A129
  constraint concentric A129 A130
  constraint concentric A130 A131
  constraint concentric A131 A132
  constraint concentric A132 A133
  constraint concentric A133 A134
  constraint concentric A134 A135
  constraint concentric A135 A136
  constraint concentric A136 A137
  constraint concentric A137 A138
  constraint concentric A138 A139
  constraint concentric A139 A140
  constraint concentric A140 A141
  constraint concentric A141 A142
  constraint concentric A142 A143
  constraint concentric A143 A144
  constraint concentric A144 A145
  constraint collinear L114 L130
  constraint collinear L115 L130
  constraint collinear L116 L130
  constraint collinear L117 L130
  constraint collinear L118 L130
  constraint collinear L119 L130
  constraint collinear L120 L130
  constraint collinear L121 L130
  constraint collinear L122 L130
  constraint collinear L123 L130
  constraint collinear L124 L130
  constraint collinear L125 L130
  constraint collinear L126 L130
  constraint collinear L127 L130
  constraint collinear L128 L130
  constraint collinear L129 L130
  constraint collinear L130 L131
  constraint concentric A134 A146
  constraint tangent A147 A148
  constraint tangent A148 A149
  constraint tangent A149 A150
  constraint tangent A147 A150
  constraint coincident A110.centre A111.centre
  constraint coincident A51 A162.end
  constraint coincident A48 A162.start
  constraint horizontal A37.start L40.end
  constraint horizontal L40.end A36.end
  constraint midpoint L40.start L41
  constraint coincident P121 P120
  constraint coincident A166 A193.start
  constraint concentric A193 A194
  constraint coincident A168 A194.start
  constraint concentric A194 A195
  constraint coincident A170 A195.start
  constraint concentric A195 A196
  constraint coincident A172 A196.start
  constraint concentric A196 A197
  constraint coincident A174 A197.start
  constraint concentric A197 A198
  constraint coincident A176 A198.start
  constraint concentric A198 A199
  constraint coincident A178 A199.start
  constraint concentric A199 A200
  constraint coincident A180 A200.start
  constraint concentric A200 A201
  constraint coincident A182 A201.start
  constraint concentric A201 A202
  constraint coincident A184 A202.start
  constraint concentric A202 A203
  constraint coincident A186 A203.start
  constraint concentric A203 A204
  constraint coincident A188 A204.start
  constraint concentric A204 A205
  constraint coincident A190 A205.start
  constraint concentric A205 A206
  constraint coincident A192 A206.start
  constraint concentric A206 A207
  constraint coincident A36 A207.start
  constraint concentric A207 A208
  constraint coincident A164 A208.start
  constraint tangent A209 A210
  constraint tangent A210 A211
  constraint tangent A211 A212
  constraint tangent A209 A212
  measures "d2" distance of L0 L130
  measures "d3" distance of L4 L130
  measures "d4" distance of L1 L2
  measures "d5" radius of A0
  measures "d6" distance of A0.start L4.end
  measures "d12" distance of A37.end A36.start
  measures "d14" radius of A36
  measures "d16" distance of L40.end L40.start
  measures "d19" diameter of A111
  measures "d20" radius of A38
  measures "d21" radius of A39
  measures "d22" distance of L43.end L43.start
  measures "d23" distance of L42.end L42.start
  measures "d38" diameter of A146
  measures "d92" distance of L40.end P121
  measures "d97" diameter of A224
extrude "Extrude1" add sketch "Sketch1" along normal blind 20 contours L0 L1 L2 A0 L4 A1 L6 A2 A3 L8 A4 A5 L10 A6 A7 L12 A8 A9 L14 A10 A11 L16 A12 A13 L18 A14 A15 L20 A16 A17 L22 A18 A19 L24 A20 A21 L26 A22 A23 L28 A24 A25 L30 A26 A27 L32 A28 A29 L34 A30 A31 L36 A32 A33 L38 A34 A35 L114 L115 L116 L117 L118 L119 L120 L121 L122 L123 L124 L125 L126 L127 L128 L129 L130 L131 makes body 1
sketch "Sketch2" plane through (0, 0, 0) normal (0, 1, 0) x (1, 0, 0)
  line L0 (22, -6) -> (22, 4)
  line L1 (22, 4) -> (-2, 4)
  line L2 (-2, 4) -> (-2, -6)
  line L3 (0, -10) -> (0, 0)
  line L4 (0, 0) -> (20, 0)
  line L5 (20, 0) -> (20, -10)
  line L6 (-2, -6) -> (0, -6)
  line L7 (20, -6) -> (22, -6)
  dimension "d46" = 24
  dimension "d47" = 10
  dimension "d48" = 2
  dimension "d49" = 4
  constraint horizontal L6
  constraint vertical L0
  constraint horizontal L1
  constraint vertical L2
  constraint coincident L3 L6.end
  constraint coincident L5 L7.start
  constraint collinear L6 L7
  measures "d46" distance of L0 L2
  measures "d47" distance of L1 L7
  measures "d48" distance of L0 L5
  measures "d49" distance of L1 L4
extrude "Extrude6" add sketch "Sketch2" along normal blind 360 separate body makes body 2
copy_body "Body->Comp1" bodies 1 removing the originals makes body 3 in component "Rack gear"
copy_body "Body->Comp6" bodies 2 removing the originals makes body 4 in component "Rack"
component "Rack gear" placed x (1, 0, 0) y (0, 1, 0) z (0, 0, 1) at (22.9777, 271.6631, 49.4511)
component "Rack" placed x (1, 0, 0) y (0, 1, 0) z (0, 0, 1) at (0, 132, 14)
